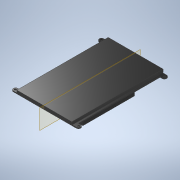
# Autodesk Inventor part: Display_EVICIV7Inch
Saved by Autodesk Inventor 2021.3 (Build 253353000, 353)
## iProperties
Created: 2021-05-26
Part Number: Display_EVICIV7Inch
Material: 一般
Document SubType Name: Modeling
Designer: gisen
Density: 1 g/cm^3
Appearance: 光沢 - 黒
Author: gisen
Autodesk Inventor part; units mm, degrees
ref_plane "YZ Plane" through (0, 0, 0) normal (1, 0, 0) x (0, 1, 0)
ref_plane "XZ Plane" through (0, 0, 0) normal (0, 1, 0) x (-1, 0, 0)
ref_plane "XY Plane" through (0, 0, 0) normal (0, 0, 1) x (1, 0, 0)
sketch "スケッチ1" plane through (0, 0, 0) normal (0, 1, 0) x (-1, 0, 0)
  line L0 (0, 0) -> (107, 0)
  line L1 (107, 0) -> (107, -165)
  line L2 (107, -165) -> (0, -165)
  line L3 (0, -165) -> (0, 0)
  line L4 (107, 0) -> (114.96, 0)
  line L5 (114.96, 0) -> (114.96, -8)
  line L6 (114.96, -8) -> (107, -8)
  line L7 (107, -8) -> (107, 0)
  line L8 (53.5, 0) -> (53.5, -165)
  circle A0 centre (111.35, -4) radius 1.75
  line L9 (107, -82.5) -> (0, -82.5)
  circle A1 centre (110.96, -4) radius 4
  line L10 (107, -165) -> (114.96, -165)
  line L11 (114.96, -157) -> (107, -157)
  circle A2 centre (111.35, -161) radius 1.75
  circle A3 centre (110.96, -161) radius 4
  line L12 (0, 0) -> (-7.96, 0)
  line L13 (-7.96, -8) -> (0, -8)
  circle A4 centre (-4.35, -4) radius 1.75
  circle A5 centre (-3.96, -4) radius 4
  circle A6 centre (-3.96, -161) radius 4
  circle A7 centre (-4.35, -161) radius 1.75
  line L14 (-7.96, -157) -> (0, -157)
  line L15 (0, -165) -> (-7.96, -165)
  point P0 (109.6, -4)
  point P1 (110.96, -8)
  point P2 (110.96, 0)
  point P3 (-3.96, 0)
  point P4 (-3.96, -8)
  point P5 (-3.96, -157)
  point P6 (-3.96, -165)
  point P7 (110.96, -165)
  point P8 (110.96, -157)
  point P9 (0, -4.5643)
  point P10 (0, -3.4357)
  point P11 (107, -4.5643)
  point P12 (107, -3.4357)
  dimension "d6" = 3.5
  dimension "d0" = 107
  dimension "d1" = 165
  dimension "d2" = 8
  dimension "d3" = 7.96
  dimension "d5" = 56.1
  dimension "d7" = 8
  constraints: 32 end point, 15 symmetric about line, 7 centre point, 4 midpoint, 4 parallel, 2 horizontal, 2 perpendicular, 1 horizontal alignment, 1 tangent, 8 other
  measures "d0" distance of L0.start L0.end
  measures "d1" distance of L0.end L1.end
  measures "d2" distance of L4.end L5.end
  measures "d3" distance of L0.end L4.end
  measures "d5" distance from line of L8 point (109.6, -4)
  measures "d7" diameter of A1
extrude "押し出し1" add sketch "スケッチ1" along normal blind 1.7 contours L0 L8 L9 L3 A5 | L3 A5 L12 | L0 L1 A1 L9 L8 | A5 L3 | L3 A5 | L4 A1 L1 | L9 L1 A3 L2 L8 | L8 L2 L3 A6 L9 | L3 L13 A5 | A1 L1 | L1 A1 | A1 L6 L1 | L1 A3 L10 | L15 A6 L3 | L11 A3 L1 | L3 A6 L14 | A3 L1 | L1 A3 | A6 L3 | L3 A6
sketch "スケッチ2" plane through (0, 1.7, 0) normal (0, 1, 0) x (1, 0, 0)
  arc A0 (-110.96, 8) -> (-110.96, 0) centre (-110.96, 4) ccw projected
  line L0 (-110.96, 0) -> (3.96, 0) projected
  arc A1 (3.96, 0) -> (3.96, 8) centre (3.96, 4) ccw projected
  line L1 (3.96, 8) -> (0, 8) projected
  line L2 (0, 8) -> (0, 157) projected
  line L3 (0, 157) -> (3.96, 157) projected
  arc A2 (3.96, 157) -> (3.96, 165) centre (3.96, 161) ccw projected
  line L4 (3.96, 165) -> (-110.96, 165) projected
  arc A3 (-110.96, 165) -> (-110.96, 157) centre (-110.96, 161) ccw projected
  line L5 (-110.96, 157) -> (-107, 157) projected
  line L6 (-107, 157) -> (-107, 8) projected
  line L7 (-107, 8) -> (-110.96, 8) projected
  circle A4 centre (4.35, 161) radius 1.75 projected
  circle A5 centre (4.35, 4) radius 1.75 projected
  circle A6 centre (-111.35, 161) radius 1.75 projected
  circle A7 centre (-111.35, 4) radius 1.75 projected
  line L8 (-103.65, -0.9) -> (-3.35, -0.9)
  line L9 (-3.35, -0.9) -> (-3.35, 165.9)
  line L10 (-3.35, 165.9) -> (-103.65, 165.9)
  line L11 (-103.65, 165.9) -> (-103.65, -0.9)
  line L12 (-103.65, -0.9) -> (-3.35, 165.9) construction
  line L13 (-3.35, -0.9) -> (-103.65, 165.9) construction
  point P0 (0, 0)
  point P1 (-53.5, 82.5)
  dimension "d10" = 100.3
  dimension "d11" = 53.5
  dimension "d12" = 82.5
  dimension "d13" = 166.8
  constraints: 12 end point, 2 midpoint, 2 parallel, 1 horizontal, 1 perpendicular
  measures "d10" distance of L8.start L8.end
  measures "d11" distance from line of L2 point (-53.5, 82.5)
  measures "d12" distance from line of L0 point (-53.5, 82.5)
  measures "d13" distance of L8.end L9.end
extrude "押し出し2" add sketch "スケッチ2" along normal blind 5.3 contours L11 L4 L9 L0 | L0 L9 L8 L11 | L11 L10 L9 L4
sketch "スケッチ3" plane through (0, 0, 0) normal (0, -1, 0) x (1, 0, 0)
  arc A0 (-110.96, 0) -> (-110.96, -8) centre (-110.96, -4) ccw projected
  line L0 (-107, -8) -> (-110.96, -8) projected
  line L1 (-107, -157) -> (-107, -8) projected
  line L2 (-110.96, -157) -> (-107, -157) projected
  arc A1 (-110.96, -157) -> (-110.96, -165) centre (-110.96, -161) ccw projected
  line L3 (3.96, -165) -> (-110.96, -165) projected
  arc A2 (3.96, -165) -> (3.96, -157) centre (3.96, -161) ccw projected
  line L4 (0, -157) -> (3.96, -157) projected
  line L5 (0, -8) -> (0, -157) projected
  line L6 (3.96, -8) -> (0, -8) projected
  arc A3 (3.96, -8) -> (3.96, 0) centre (3.96, -4) ccw projected
  line L7 (-110.96, 0) -> (3.96, 0) projected
  circle A4 centre (4.35, -161) radius 1.75 projected
  circle A5 centre (4.35, -4) radius 1.75 projected
  circle A6 centre (-111.35, -161) radius 1.75 projected
  circle A7 centre (-111.35, -4) radius 1.75 projected
  line L8 (-89, -36) -> (-20, -36)
  line L9 (-20, -36) -> (-20, -130)
  line L10 (-20, -130) -> (-89, -130)
  line L11 (-89, -130) -> (-89, -36)
  circle A8 centre (-23.5, -39.5) radius 1.75
  line L12 (-20, -83) -> (-89, -83)
  line L13 (-54.5, -130) -> (-54.5, -36)
  circle A9 centre (-23.5, -126.5) radius 1.75
  circle A10 centre (-85.5, -39.5) radius 1.75
  circle A11 centre (-85.5, -126.5) radius 1.75
  point P0 (0, 0)
  point P1 (-54.5, -83)
  dimension "d16" = 94
  dimension "d17" = 69
  dimension "d18" = 36
  dimension "d19" = 20
  dimension "d22" = 34.5
  dimension "d23" = 47
  dimension "d24" = 3.5
  dimension "d25" = 3.5
  dimension "d26" = 3.5
  constraints: 12 end point, 4 centre point, 4 midpoint, 3 symmetric about line, 2 parallel, 1 horizontal, 1 perpendicular, 3 other
  measures "d16" distance of L8.end L9.end
  measures "d17" distance of L9.end L10.end
  measures "d18" distance between parallel lines of L7 L8
  measures "d19" distance between parallel lines of L5 L9
  measures "d22" distance from line of L11 point (-54.5, -83)
  measures "d23" distance from line of L10 point (-54.5, -83)
  measures "d24" diameter of A8
  measures "d25" distance from line of L9 A8.centre
  measures "d26" distance from line of L8 A8.centre
extrude "押し出し3" add sketch "スケッチ3" along normal blind 26 contours L8 L13 L12 L11 | L8 L9 L12 L13 | L12 L13 L10 L11 | L12 L9 L10 L13
ref_plane "作業平面1" through (-53.5, 1.7, 0) normal (1, 0, 0) x (0, 0, -1)
